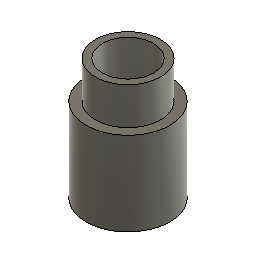
Adapter Validation Compressor Pump 11mm to 15mm (Autodesk Fusion 360 design; units mm, degrees)
Autodesk Fusion 360 part; units mm, degrees
sketch "Sketch1" plane through (0, 0, 0) normal (0, 1, 0) x (1, 0, 0)
  circle A0 centre (0, 0) radius 7.5
  circle A1 centre (0, 0) radius 9
  dimension "d1" = 15
  dimension "d2" = 1.5
  constraint coincident A0.centre A1.centre
  measures "d1" diameter of A0
  measures "d2" distance of A0 A1
extrude "Extrude1" add sketch "Sketch1" along normal blind 16 makes body 1
ref_plane "WorkPlane1" through (0, 16, 0) normal (0, 1, 0) x (1, 0, 0)
sketch "Sketch2" plane through (0, 16, 0) normal (0, 1, 0) x (1, 0, 0)
  circle A0 centre (0, 0) radius 9
  circle A1 centre (0, 0) radius 9
  constraint coincident A0.centre A1.centre
  constraint tangent A0 A1
extrude "Extrude2" add sketch "Sketch2" along normal blind 2 bodies 1
ref_plane "WorkPlane2" through (0, 18, 0) normal (0, 1, 0) x (1, 0, 0)
sketch "Sketch3" plane through (0, 18, 0) normal (0, 1, 0) x (1, 0, 0)
  circle A0 centre (0, 0) radius 5.5
  circle A1 centre (0, 0) radius 7
  dimension "d9" = 11
  dimension "d10" = 1.5
  constraint coincident A0.centre A1.centre
  constraint concentric A0 A1
  measures "d9" diameter of A0
  measures "d10" distance of A0 A1
extrude "Extrude3" add sketch "Sketch3" along normal blind 8 bodies 1
extrude "Extrude4" cut 1 faces at (-1.4907, 18, -0.2732) along direction (0, -1, 0) blind 2 on bodies 1 bodies 1
copy_body "Body->Comp1" bodies 1 removing the originals makes body 2 in component "Adapter 11-15"
component "Adapter 11-15" placed x (1, 0, 0) y (0, 1, 0) z (0, 0, 1) at (0, 0, 0)
